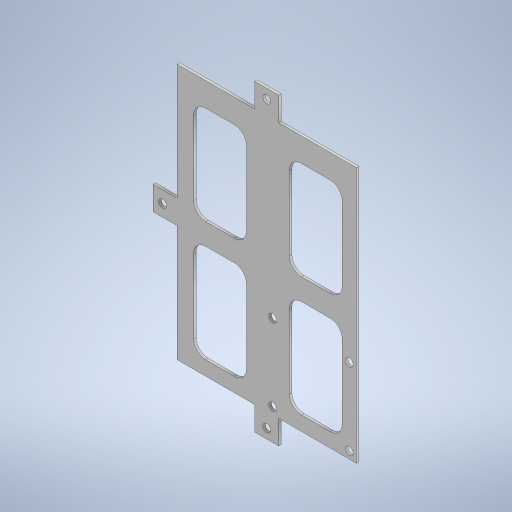
# Autodesk Inventor part: PCB_board_box_right
Saved by Autodesk Inventor 2023 (Build 270158000, 158)
## iProperties
Created: 2023-05-25
Part Number: PCB_board_box_right
Material: 一般
Document SubType Name: Sheet Metal
Designer: 310611102
Density: 1 g/cm^3
Sheet Metal Rule: Default_mm
Appearance: 預設
Author: 310611102
Autodesk Inventor part; units mm, degrees
ref_plane "YZ Plane" through (0, 0, 0) normal (1, 0, 0) x (0, 1, 0)
ref_plane "XZ Plane" through (0, 0, 0) normal (0, 1, 0) x (-1, 0, 0)
ref_plane "XY Plane" through (0, 0, 0) normal (0, 0, 1) x (1, 0, 0)
sketch "Sketch1" plane through (0, 0, 0) normal (0, 0, 1) x (1, 0, 0)
  line L0 (-37.5, 53.5) -> (37.5, 53.5)
  line L1 (37.5, 53.5) -> (37.5, -53.5)
  line L2 (37.5, -53.5) -> (-37.5, -53.5)
  line L3 (-37.5, -53.5) -> (-37.5, 53.5)
  line L4 (-37.5, 53.5) -> (37.5, -53.5) construction
  line L5 (37.5, 53.5) -> (-37.5, -53.5) construction
  line L6 (-25.5, 43.5) -> (-13.5, 43.5)
  line L7 (-8.5, 38.5) -> (-8.5, 7.5)
  line L8 (-13.5, 2.5) -> (-25.5, 2.5)
  line L9 (-30.5, 7.5) -> (-30.5, 38.5)
  line L10 (-30.5, 43.5) -> (-8.5, 2.5) construction
  line L11 (-8.5, 43.5) -> (-30.5, 2.5) construction
  arc A0 (-25.5, 43.5) -> (-30.5, 38.5) centre (-25.5, 38.5) ccw
  arc A1 (-8.5, 38.5) -> (-13.5, 43.5) centre (-13.5, 38.5) ccw
  arc A2 (-13.5, 2.5) -> (-8.5, 7.5) centre (-13.5, 7.5) ccw
  arc A3 (-30.5, 7.5) -> (-25.5, 2.5) centre (-25.5, 7.5) ccw
  line L12 (9.5, 7.5) -> (9.5, 38.5)
  arc A4 (26.5, 2.5) -> (31.5, 7.5) centre (26.5, 7.5) ccw
  arc A5 (14.5, 43.5) -> (9.5, 38.5) centre (14.5, 38.5) ccw
  arc A6 (31.5, 38.5) -> (26.5, 43.5) centre (26.5, 38.5) ccw
  arc A7 (9.5, 7.5) -> (14.5, 2.5) centre (14.5, 7.5) ccw
  line L13 (26.5, 2.5) -> (14.5, 2.5)
  line L14 (31.5, 38.5) -> (31.5, 7.5)
  line L15 (9.5, 43.5) -> (31.5, 2.5) construction
  line L16 (14.5, 43.5) -> (26.5, 43.5)
  line L17 (31.5, 43.5) -> (9.5, 2.5) construction
  line L18 (-30.5, -42.5) -> (-30.5, -11.5)
  arc A8 (-13.5, -47.5) -> (-8.5, -42.5) centre (-13.5, -42.5) ccw
  arc A9 (-25.5, -6.5) -> (-30.5, -11.5) centre (-25.5, -11.5) ccw
  arc A10 (-8.5, -11.5) -> (-13.5, -6.5) centre (-13.5, -11.5) ccw
  arc A11 (-30.5, -42.5) -> (-25.5, -47.5) centre (-25.5, -42.5) ccw
  line L19 (-13.5, -47.5) -> (-25.5, -47.5)
  line L20 (-8.5, -11.5) -> (-8.5, -42.5)
  line L21 (-30.5, -6.5) -> (-8.5, -47.5) construction
  line L22 (-25.5, -6.5) -> (-13.5, -6.5)
  line L23 (-8.5, -6.5) -> (-30.5, -47.5) construction
  line L24 (9.5, -42.5) -> (9.5, -11.5)
  arc A12 (26.5, -47.5) -> (31.5, -42.5) centre (26.5, -42.5) ccw
  arc A13 (14.5, -6.5) -> (9.5, -11.5) centre (14.5, -11.5) ccw
  arc A14 (31.5, -11.5) -> (26.5, -6.5) centre (26.5, -11.5) ccw
  arc A15 (9.5, -42.5) -> (14.5, -47.5) centre (14.5, -42.5) ccw
  line L25 (26.5, -47.5) -> (14.5, -47.5)
  line L26 (31.5, -11.5) -> (31.5, -42.5)
  line L27 (9.5, -6.5) -> (31.5, -47.5) construction
  line L28 (14.5, -6.5) -> (26.5, -6.5)
  line L29 (31.5, -6.5) -> (9.5, -47.5) construction
  line L30 (0, 0) -> (0, 8.3009)
  line L31 (0, 0) -> (4.4939, 0)
  point P0 (-19.5, 23)
  point P1 (20.5, 23)
  point P2 (-19.5, -27)
  point P3 (20.5, -27)
  dimension "d0" = 107
  dimension "d1" = 75
  dimension "d3" = 22
  dimension "d4" = 41
  dimension "d5" = 5
  dimension "d8" = 40
  dimension "d11" = 50
  dimension "d14" = 10
  dimension "d15" = 7
  measures "d0" distance of L0.end L1.end
  measures "d1" distance of L0.start L0.end
  measures "d3" distance of L10.start L11.start
  measures "d4" distance of L11.end L10.start
  measures "d5" radius of A0
  measures "d8" distance of L9.start L12.start
  measures "d11" distance of L9.start L18.start
  measures "d14" distance between parallel lines of L0 L6
  measures "d15" distance between parallel lines of L3 L9
extrude "Plate1" add sketch "Sketch1" along normal blind 1
sketch "Sketch2" plane through (0, 0, 1) normal (0, 0, 1) x (1, 0, 0)
  line L0 (37.5, 53.5) -> (37.5, -53.5)
  line L1 (-37.5, -53.5) -> (-37.5, 53.5)
  line L2 (-47.5, 5) -> (-37.5, 5)
  line L3 (-37.5, 5) -> (-37.5, -5)
  line L4 (-37.5, -5) -> (-47.5, -5)
  line L5 (-47.5, -5) -> (-47.5, 5)
  line L6 (-47.5, 5) -> (-37.5, -5) construction
  line L7 (-37.5, 5) -> (-47.5, -5) construction
  line L8 (-37.5, 53.5) -> (37.5, 53.5)
  line L9 (-5, 63.5) -> (5, 63.5)
  line L10 (5, 63.5) -> (5, 53.5)
  line L11 (5, 53.5) -> (-5, 53.5)
  line L12 (-5, 53.5) -> (-5, 63.5)
  line L13 (-5, 63.5) -> (5, 53.5) construction
  line L14 (5, 63.5) -> (-5, 53.5) construction
  line L15 (0, 0) -> (10.0151, 0)
  line L16 (-5, -63.5) -> (5, -63.5)
  line L17 (5, -63.5) -> (5, -53.5)
  line L18 (5, -53.5) -> (-5, -53.5)
  line L19 (-5, -53.5) -> (-5, -63.5)
  line L20 (-5, -63.5) -> (5, -53.5) construction
  line L21 (5, -63.5) -> (-5, -53.5) construction
  circle A0 centre (0, 59.5) radius 1.6
  circle A1 centre (-43.5, 0) radius 1.6
  circle A2 centre (0, -59.5) radius 1.6
  point P0 (-42.5, 0)
  point P1 (0, 58.5)
  point P2 (0, -58.5)
  point P3 (37.5, 38.5)
  dimension "d23" = 10
  dimension "d24" = 10
  dimension "d27" = 10
  dimension "d28" = 10
  dimension "d43" = 3.2
  dimension "d44" = 3.2
  dimension "d45" = 4
  dimension "d46" = 4
  measures "d23" distance of L9.start L9.end
  measures "d24" distance of L9.end L10.end
  measures "d27" distance of L2.start L2.end
  measures "d28" distance of L4.end L2.start
  measures "d43" diameter of A0
  measures "d44" diameter of A1
  measures "d45" distance from line of L5 A1.centre
  measures "d46" distance from line of L9 A0.centre
sheet face with bend "Face2" sketch "Sketch2" thickness 1 toward (0, 0, -1) bend radius 1 relief straight relief width 1 relief depth 0.5
bend "Bend1"
sketch "Sketch3" plane through (0, 0, 1) normal (0, 0, 1) x (1, 0, 0)
  circle A0 centre (2.5, -18.5) radius 1.6
  line L0 (2.5, -18.5) -> (11.3604, -18.5)
  line L1 (2.5, -18.5) -> (2.5, -34.5603)
  circle A1 centre (34.5, -18.5) radius 1.6
  circle A2 centre (2.5, -50.5) radius 1.6
  circle A3 centre (34.5, -50.5) radius 1.6
  line L2 (37.5, 53.5) -> (37.5, -53.5) projected
  line L3 (37.5, -53.5) -> (5, -53.5) projected
  point P0 (0, 0)
  dimension "d48" = 3.2
  dimension "d51" = 32
  dimension "d54" = 32
  dimension "d57" = 35
  dimension "d58" = 35
  constraints: 4 centre point, 4 end point, 2 horizontal, 2 vertical, 6 other
  measures "d48" diameter of A0
  measures "d51" distance of L0.start A1.centre
  measures "d54" distance of L0.start A2.centre
  measures "d57" distance from line of L2 L0.start
  measures "d58" distance from line of L3 L0.start
extrude "Cut1" cut sketch "Sketch3" against normal blind 1
equation "\"d59\" = 厚度"
equation "\"d2\" = 厚度"
equation "\"d37\" = 折彎半徑"
equation "\"d38\" = 折彎離隙寬度"
equation "\"d40\" = 最小剩餘"
equation "\"d39\" = 折彎離隙深度"
equation "\"d41\" = 轉移半徑"
equation "\"折彎半徑\" = 厚度"
equation "\"折彎離隙寬度\" = 厚度"
equation "\"折彎離隙深度\" = 0.5 * 厚度"
equation "\"轉角離隙大小\" = 4 * 厚度"
equation "\"最小剩餘\" = 2 * 厚度"
equation "\"轉移半徑\" = 折彎半徑"
equation "\"Jacobi半徑大小\" = 折彎半徑"
equation "\"間隙大小\" = 厚度"
equation "\"厚度\" = 1"
body "Solid1"
